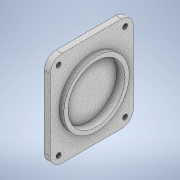
# Autodesk Inventor part: Deckel Endewelle
Saved by Autodesk Inventor 2022 (Build 260153000, 153)
## iProperties
Created: 2023-01-28
Part Number: Deckel Endewelle
Material: Aluminium 6061
Document SubType Name: Modeling
Designer: Matias Nicky
Density: 2.7 g/cm^3
Appearance: Aluminiumguss
Author: Matias Nicky
Autodesk Inventor part; units mm, degrees
ref_plane "YZ Plane" through (0, 0, 0) normal (1, 0, 0) x (0, 1, 0)
ref_plane "XZ Plane" through (0, 0, 0) normal (0, 1, 0) x (-1, 0, 0)
ref_plane "XY Plane" through (0, 0, 0) normal (0, 0, 1) x (1, 0, 0)
sketch "Skizze1" plane through (0, 0, 0) normal (1, 0, 0) x (0, 1, 0)
  line L0 (-43, 62) -> (37, 62)
  line L1 (37, 62) -> (37, -8)
  line L2 (37, -8) -> (-43, -8)
  line L3 (-43, -8) -> (-43, 62)
  line L4 (-43, 62) -> (37, -8) construction
  line L5 (37, 62) -> (-43, -8) construction
  point P0 (-3, 27)
  dimension "d3" = 80
  dimension "d4" = 70
  constraints: 12 end point, 2 midpoint, 2 parallel, 1 horizontal, 1 perpendicular
  measures "d3" distance of L1.end L2.end
  measures "d4" distance between parallel lines of L2 L0
extrude "Extrusion1" add sketch "Skizze1" along normal blind 5
sketch "Skizze2" plane through (5, 0, 0) normal (1, 0, 0) x (0, 0, -1)
  circle A0 centre (-27, -3) radius 27.5
  line L0 (8, 37) -> (-62, 37) projected
  line L1 (-62, 37) -> (-62, -43) projected
  point P0 (0, 0)
  dimension "d5" = 55
  dimension "d11" = 40
  dimension "d12" = 35
  constraints: 1 centre point
  measures "d5" diameter of A0
  measures "d11" distance from line of L0 A0.centre
  measures "d12" distance from line of L1 A0.centre
extrude "Extrusion2" add sketch "Skizze2" along normal blind 4
sketch "Skizze3" plane through (9, -3, 27) normal (1, 0, 0) x (0, 0, -1)
  circle A0 centre (0, 0) radius 24
  point P0 (27, 3)
  dimension "d8" = 48
  constraints: 1 centre point
  measures "d8" diameter of A0
extrude "Extrusion3" cut sketch "Skizze3" against normal through all
fillet "Rundung1" radius 10 4 edges at (2.5, 37, -8) (2.5, 37, 62) (2.5, -43, 62) (2.5, -43, -8)
sketch "Skizze4" plane through (5, 0, 0) normal (1, 0, 0) x (0, 0, -1)
  circle A0 centre (-27, -3) radius 33.55
  line L0 (-2, 37) -> (-52, 37) projected
  line L1 (-62, 27) -> (-62, -33) projected
  line L2 (8, -33) -> (8, 27) projected
  line L3 (-52, -43) -> (-2, -43) projected
  point P0 (0, 0)
  point P1 (-55, 30)
  point P2 (1, 30)
  point P3 (1, -36)
  point P4 (-55, -36)
  dimension "d14" = 67.1
  dimension "d15" = 7
  dimension "d16" = 7
  dimension "d17" = 7
  dimension "d18" = 7
  dimension "d19" = 7
  dimension "d20" = 7
  dimension "d21" = 7
  dimension "d29" = 7
  constraints: 1 centre point, 1 coincident
  measures "d14" diameter of A0
  measures "d15" distance from line of L0 point (-55, 30)
  measures "d16" distance from line of L1 point (-55, 30)
  measures "d17" distance from line of L0 point (1, 30)
  measures "d18" distance from line of point (1, 30) L2
  measures "d19" distance from line of L2 point (1, -36)
  measures "d20" distance from line of L3 point (-55, -36)
  measures "d21" distance from line of point (-55, -36) L1
  measures "d29" distance from line of L3 point (1, -36)
hole "Bohrung1" at (5, 30, 55) at (5, 30, -1) at (5, -36, -1) at (5, -36, 55) direction (-1, 0, 0) diameter 4.134 end through all thread size "M5x0.8" class "6H" standard "ANSI Metric M Profile"
sketch "Skizze5" plane through (0, 0, 0) normal (-1, 0, 0) x (0, 0, 1)
  circle A0 centre (27, -3) radius 24 projected
  circle A1 centre (27, -3) radius 27.5
  circle A2 centre (27, -3) radius 10
  point P0 (0, 0)
  dimension "d30" = 55
  dimension "d39" = 20
  constraints: 2 centre point, 2 coincident
  measures "d30" diameter of A1
  measures "d39" diameter of A2
extrude "Extrusion5" add sketch "Skizze5" along normal mid plane 4 contours A0 | A1 | A2
